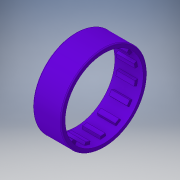
# Autodesk Inventor part: TP Tire
Saved by Autodesk Inventor 2018 (Build 220112000, 112)
## iProperties
Created: 2018-02-18
Part Number: TP Tire
Material: Rubber, Silicone
Document SubType Name: Modeling
Designer: Blue Mist
Density: 1.25 g/cm^3
Appearance: Rubber - Black
Author: Blue Mist
Autodesk Inventor part; units mm, degrees
note: some values were not read from the file. Chosen so that the rebuilt part matches the saved one: arc direction of "Extrusion2".
ref_plane "YZ Plane" through (0, 0, 0) normal (1, 0, 0) x (0, 1, 0)
ref_plane "XZ Plane" through (0, 0, 0) normal (0, 1, 0) x (-1, 0, 0)
ref_plane "XY Plane" through (0, 0, 0) normal (0, 0, 1) x (1, 0, 0)
sketch "Sketch1" plane through (0, 0, 0) normal (0, 0, 1) x (1, 0, 0)
  line L0 (0, 0) -> (0, 19.6088) construction
  line L1 (0, 19.6088) -> (14.224, 19.6088)
  line L2 (14.224, 19.6088) -> (14.224, 21.1328)
  line L3 (13.716, 21.6408) -> (0.508, 21.6408)
  line L4 (0, 21.1328) -> (0, 19.6088)
  arc A0 (14.224, 21.1328) -> (13.716, 21.6408) centre (13.716, 21.1328) ccw
  arc A1 (0.508, 21.6408) -> (0, 21.1328) centre (0.508, 21.1328) ccw
  line L5 (-2.9921, 0) -> (17.2161, 0) projected
  point P0 (14.224, 21.6408)
  point P1 (0, 21.6408)
  dimension "d0" = 19.6088
  dimension "d1" = 14.224
  dimension "d2" = 2.032
  dimension "d3" = 0.508
  constraints: 10 end point, 5 point on line, 4 perpendicular, 4 point on circle, 4 tangent, 2 centre point, 1 equal radius, 1 vertical
  measures "d0" distance of L0.start L0.end
  measures "d1" distance of L0.end L1.end
  measures "d2" distance of L1.end point (14.224, 21.641)
  measures "d3" radius of A0
revolve "Revolution1" add sketch "Sketch1" angle 360 about axis through (-10, 0, 0) along (1, 0, 0)
sketch "Sketch2" plane through (0, 0, 0) normal (0, 1, 0) x (-1, 0, 0)
  line L0 (0, 19.6088) -> (0, -19.6088) projected
  line L1 (-14.224, 19.6088) -> (-14.224, -19.6088) projected
  line L2 (-14.224, -19.6088) -> (0, -19.6088) projected
  line L3 (-14.224, 19.6088) -> (-14.224, -19.6088) projected
  line L4 (0, 19.6088) -> (0, -19.6088) projected
  line L5 (-2.54, 0) -> (-11.684, 0)
  line L6 (-11.684, 0) -> (-11.684, -19.6088)
  line L7 (-2.54, 0) -> (-2.54, -19.6088)
  line L8 (2.8448, 0) -> (-17.0688, 0) projected
  point P0 (0, 0)
  dimension "d5" = 2.54
  dimension "d6" = 2.54
  constraints: 6 end point, 2 perpendicular, 2 point on line, 1 horizontal
  measures "d5" distance from line of L0 L5.start
  measures "d6" distance from line of L1 L5.end
revolve "Revolution2" add sketch "Sketch2" angle 360 about axis through (-10, 0, 0) along (1, 0, 0) contours L7 L2 L6 L5
sketch "Sketch3" plane through (2.54, 0, 0) normal (-1, 0, 0) x (0, 0, 1)
  circle A0 centre (0, 0) radius 18.2245
  dimension "d8" = 36.449
  constraints: 1 centre point, 1 coincident
  measures "d8" diameter of A0
extrude "Extrusion1" cut sketch "Sketch3" against normal blind 25.4
sketch "Sketch4" plane through (2.54, 0, 0) normal (-1, 0, 0) x (0, 0, 1)
  circle A0 centre (0, 0) radius 19.6088 projected
  circle A1 centre (0, 0) radius 18.2245 projected
  arc A2 (-18.0283, 2.667) -> (-18.0283, -2.667) centre (0, 0) ccw
  arc A3 (-19.4266, 2.667) -> (-19.4266, -2.667) centre (0, 0) ccw
  line L0 (-18.0283, -2.667) -> (-19.4266, -2.667)
  line L1 (-18.0283, 2.667) -> (-19.4266, 2.667)
  point P0 (-16.0023, 2.667)
  point P1 (-16.0023, -2.667)
  point P2 (-17.1751, -2.667)
  point P3 (-17.1751, 2.667)
  constraints: 9 point on circle, 4 end point, 2 centre point, 1 concentric, 1 horizontal
extrude "Extrusion2" cut sketch "Sketch4" against normal blind 25.4 contours L1 A1 L0 A0 picked at (-18.5525, 2.0753)
pattern_circular "Circular Pattern1" count 15 over 360 about axis through (-10, 0, 0) along (1, 0, 0) of "Extrusion2"
body "Solid1"
